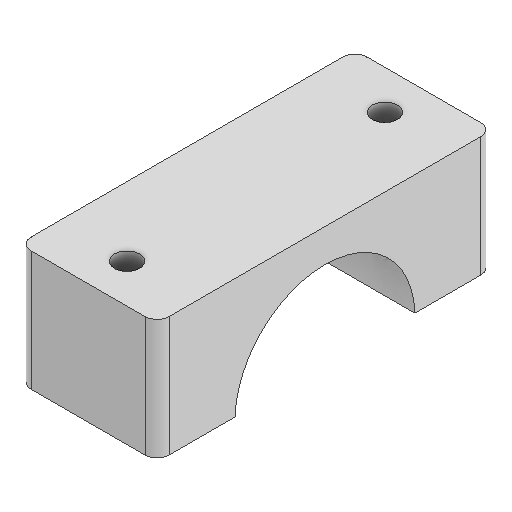
# Autodesk Inventor part: 3DP_ASA_Preamp_Case_Clamp
Saved by Autodesk Inventor 2026.1 (Build 301233000, 233)
## iProperties
Created: 2025-06-27
Part Number: 3DP_ASA_Preamp_Case_Clamp
Material: Generic
Document SubType Name: Modeling
Designer: User
Density: 1 g/cm^3
Appearance: Default
Author: User
Autodesk Inventor part; units mm, degrees
ref_plane "YZ Plane" through (0, 0, 0) normal (1, 0, 0) x (0, 1, 0)
ref_plane "XZ Plane" through (0, 0, 0) normal (0, 1, 0) x (-1, 0, 0)
ref_plane "XY Plane" through (0, 0, 0) normal (0, 0, 1) x (1, 0, 0)
sketch "Sketch1" plane through (0, 0, 0) normal (0, 1, 0) x (-1, 0, 0)
  line L0 (12.5, 25.5) -> (-12.5, 25.5)
  line L1 (-12.5, 25.5) -> (-12.5, -25.5)
  line L2 (-12.5, -25.5) -> (12.5, -25.5)
  line L3 (12.5, -25.5) -> (12.5, 25.5)
  line L4 (13, 26) -> (-13, 26)
  line L5 (-13, 26) -> (-13, -26)
  line L6 (-13, -26) -> (13, -26)
  line L7 (13, -26) -> (13, 26)
  line L8 (15, 28) -> (-15, 28)
  line L9 (-15, 28) -> (-15, -28)
  line L10 (-15, -28) -> (15, -28)
  circle A0 centre (8.5, 21.5) radius 2
  circle A1 centre (8.5, -21.5) radius 2
  circle A2 centre (-8.5, 21.5) radius 2
  circle A3 centre (-8.5, -21.5) radius 2
  line L11 (15, -28) -> (38, -28)
  line L12 (38, -28) -> (38, -26)
  line L13 (38, -26) -> (13, -26)
  line L14 (13, 26) -> (38, 26)
  line L15 (38, 26) -> (38, 28)
  line L16 (38, 28) -> (15, 28)
  line L17 (38, -26) -> (38, 26)
  line L18 (12.5, -15.5) -> (-12.5, -15.5)
  line L19 (12.5, 15.5) -> (-12.5, 15.5)
  line L20 (12.5, -15.5) -> (13, -15.5)
  line L21 (12.5, 15.5) -> (13, 15.5)
  line L22 (-12.5, -15.5) -> (-13, -15.5)
  line L23 (-12.5, 15.5) -> (-13, 15.5)
  point P0 (0, 0)
  dimension "d0" = 51
  dimension "d1" = 25
  dimension "d2" = 12.5
  dimension "d3" = 25.5
  dimension "d4" = 4
  dimension "d5" = 4
  dimension "d6" = 4
  dimension "d7" = 4
  dimension "d8" = 0.5
  dimension "d10" = 4
  dimension "d11" = 4
  dimension "d12" = 4
  dimension "d13" = 4
  dimension "d50" = 25
  dimension "d51" = 10
  dimension "d52" = 10
  constraints: 48 end point, 12 perpendicular, 8 point on line, 5 parallel, 4 centre point, 4 coincident, 3 horizontal, 2 horizontal alignment, 2 vertical alignment, 1 vertical, 5 other
  measures "d0" distance between parallel lines of L2 L0
  measures "d1" distance of L1.end L2.end
  measures "d2" distance from line of L3 point (0, 0)
  measures "d3" distance from line of L2 point (0, 0)
  measures "d4" distance from line of L0 point (8.5, 21.5)
  measures "d5" distance from line of L3 point (8.5, 21.5)
  measures "d6" distance from line of L1 point (-8.5, 21.5)
  measures "d7" distance from line of L2 point (8.5, -21.5)
  measures "d8" distance between parallel lines of L3 L7
  measures "d10" diameter of A0
  measures "d11" diameter of A1
  measures "d12" diameter of A2
  measures "d13" diameter of A3
  measures "d50" distance between parallel lines of L17 L7
  measures "d51" distance between parallel lines of L2 L18
  measures "d52" distance between parallel lines of L0 L19
extrude "Extrusion1" add sketch "Sketch1" against normal blind 10 contours L3 L19 L1 L0 | L0 L1 L23 L5 L4 L7 L21 L3 | L21 L7 L20 L3 | L3 L18 L1 L19 | L1 L22 L5 L23 | L20 L7 L6 L5 L22 L1 L2 L3 | L3 L2 L1 L18 | L7 L14 L17 L13 | L5 L6 L13 L12 L11 L10 L9 L8 L16 L15 L14 L4 | A0 | A1 | A2 | A3
extrude "Extrusion2" add sketch "Sketch1" along normal blind 7 contours L5 L6 L13 L12 L11 L10 L9 L8 L16 L15 L14 L4
extrude "Extrusion3" cut sketch "Sketch1" against normal blind 6 contours A0 | A1 | A2 | A3
extrude "Extrusion8" cut sketch "Sketch1" against normal blind 7 contours L21 L7 L20 L3 | L3 L18 L1 L19 | L1 L22 L5 L23 | L7 L14 L17 L13
fillet "Fillet3" radius 2 6 edges at (-13, -3.5, -15.5) (-13, -3.5, -26) (13, -3.5, -15.5) (13, -3.5, 15.5) (-13, -3.5, 15.5) (-13, -3.5, 26)
sketch "Sketch7" plane through (8.5, -6, -21.5) normal (0, 1, 0) x (1, 0, 0)
  circle A0 centre (0, 0) radius 2 projected
  circle A1 centre (-17, 0) radius 2 projected
  circle A2 centre (-17, -43) radius 2 projected
  circle A3 centre (0, -43) radius 2 projected
  point P0 (-8.5, -21.5)
extrude "Extrusion9" cut sketch "Sketch7" against normal blind 1
sketch "Sketch8" plane through (-38, -10, -28) normal (-1, 0, 0) x (0, 0, 1)
  line L0 (54, 17) -> (54, 3) projected
  line L1 (54, 3) -> (2, 3) projected
  line L2 (2, 3) -> (2, 17) projected
  line L3 (0, 17) -> (2, 17) projected
  line L4 (0, 17) -> (0, 0) projected
  line L5 (56, 0) -> (0, 0) projected
  line L6 (56, 0) -> (56, 17) projected
  line L7 (54, 17) -> (56, 17) projected
  line L8 (2, 17) -> (54, 17)
  line L9 (13.7, 17) -> (13.7, 9)
  line L10 (13.7, 9) -> (19.7, 9)
  line L11 (19.7, 9) -> (19.7, 17)
  line L12 (36.7, 17) -> (36.7, 9)
  line L13 (36.7, 9) -> (42.7, 9)
  line L14 (42.7, 9) -> (42.7, 17)
  point P0 (28, 10)
  dimension "d58" = 6
  dimension "d59" = 6
  dimension "d60" = 17
  dimension "d63" = 11.7
  dimension "d66" = 8
  constraints: 14 end point, 6 point on line, 4 perpendicular, 1 parallel, 1 vertical
  measures "d58" distance between parallel lines of L11 L9
  measures "d59" distance between parallel lines of L14 L12
  measures "d60" distance between parallel lines of L12 L11
  measures "d63" distance between parallel lines of L2 L9
  measures "d66" distance between parallel lines of L8 L10
extrude "Extrusion10" add sketch "Sketch8" against normal blind 2 contours L0 L1 L2 L8 L9 L10 L11 L12 L13 L14
fillet "Fillet4" radius 2 8 edges at (-37, -1, -14.3) (-37, -1, -8.3) (-37, -1, 8.7) (-37, -1, 14.7) (-38, -1.5, 28) (15, -1.5, 28) (15, -1.5, -28) (-38, -1.5, -28)
fillet "Fillet5" radius 2 2 edges at (-36, 0, -26) (-36, 0, 26)
sketch "Sketch10" plane through (0, -10, 0) normal (0, -1, 0) x (1, 0, 0)
  line L0 (-15, 26) -> (-34, 26) projected
  arc A0 (-34, 26) -> (-36, 24) centre (-34, 24) ccw projected
  line L1 (-36, -24) -> (-36, 24) projected
  arc A1 (-36, -24) -> (-34, -26) centre (-34, -24) ccw projected
  line L2 (-34, -26) -> (-15, -26) projected
  arc A2 (-38, -26) -> (-36, -28) centre (-36, -26) ccw projected
  line L3 (-36, -28) -> (13, -28) projected
  arc A3 (13, -28) -> (15, -26) centre (13, -26) ccw projected
  line L4 (15, -26) -> (15, 26) projected
  arc A4 (15, 26) -> (13, 28) centre (13, 26) ccw projected
  line L5 (13, 28) -> (-36, 28) projected
  arc A5 (-36, 28) -> (-38, 26) centre (-36, 26) ccw projected
  line L6 (-38, 26) -> (-38, -26) projected
  line L7 (-36, 24) -> (-36, 28)
  line L8 (-36, -24) -> (-36, -28)
  line L9 (-15, 28) -> (-15, -28)
  point P0 (0, 0)
  constraints: 6 end point, 3 point on line, 2 perpendicular, 1 tangent
extrude "Extrusion11" add sketch "Sketch10" along normal blind 20 contours L9 L2 A1 L1 A0 L0 | L0 A0 L7 L5 L9 | L9 L3 L8 A1 L2 | L1 L8 A2 L6 A5 L7
sketch "Sketch11" plane through (-38, 7, -8.3) normal (-1, 0, 0) x (0, 0, 1)
  line L0 (-17.7, -37) -> (-17.7, 0) projected
  line L1 (34.3, -37) -> (-17.7, -37) projected
  line L2 (34.3, 0) -> (34.3, -37) projected
  line L3 (34.3, 0) -> (23, 0) projected
  line L4 (23, 0) -> (23, -6) projected
  arc A0 (21, -8) -> (23, -6) centre (21, -6) ccw projected
  line L5 (21, -8) -> (19, -8) projected
  arc A1 (17, -6) -> (19, -8) centre (19, -6) ccw projected
  line L6 (17, -6) -> (17, 0) projected
  line L7 (17, 0) -> (0, 0) projected
  line L8 (0, 0) -> (0, -6) projected
  arc A2 (-2, -8) -> (0, -6) centre (-2, -6) ccw projected
  line L9 (-2, -8) -> (-4, -8) projected
  arc A3 (-6, -6) -> (-4, -8) centre (-4, -6) ccw projected
  line L10 (-6, -6) -> (-6, 0) projected
  line L11 (-17.7, 0) -> (-6, 0) projected
  arc A4 (23.2917, -37) -> (-6.6917, -37) centre (8.3, -37.5) ccw
  point P0 (8.3, -7)
  dimension "d71" = 52
  dimension "d72" = 26
  dimension "d73" = 0.5
  dimension "d74" = 30
  constraints: 2 point on circle, 2 point on line, 1 centre point, 1 coincident
  measures "d71" distance between parallel lines of L0 L2
  measures "d72" distance from line of L2 point (8.3, -37.5)
  measures "d73" distance from line of L1 point (8.3, -37.5)
  measures "d74" diameter of A4
extrude "Extrusion12" cut sketch "Sketch11" against normal through all contours A4 L1
fillet "Fillet6" radius 2 2 edges at (-15, -20, 28) (-15, -20, -28)
sketch "Sketch12" plane through (0, -30, 0) normal (0, -1, 0) x (1, 0, 0)
  arc A0 (-15, 26) -> (-17, 28) centre (-17, 26) ccw projected
  line L0 (-17, 28) -> (-36, 28) projected
  arc A1 (-36, 28) -> (-38, 26) centre (-36, 26) ccw projected
  line L1 (-38, 26) -> (-38, 14.9917) projected
  line L2 (-38, 14.9917) -> (-15, 14.9917) projected
  line L3 (-15, 14.9917) -> (-15, 26) projected
  arc A2 (-17, -28) -> (-15, -26) centre (-17, -26) ccw projected
  line L4 (-15, -26) -> (-15, -14.9917) projected
  line L5 (-15, -14.9917) -> (-38, -14.9917) projected
  line L6 (-38, -14.9917) -> (-38, -26) projected
  arc A3 (-38, -26) -> (-36, -28) centre (-36, -26) ccw projected
  line L7 (-36, -28) -> (-17, -28) projected
  point P0 (0, 0)
  point P1 (-26.5, 21.5)
  point P2 (-26.5, -21.5)
  dimension "d78" = 23
  dimension "d79" = 11.5
  dimension "d80" = 13.0083
  dimension "d81" = 6.5
  dimension "d82" = 6.5
  constraints: 1 vertical alignment
  measures "d78" distance between parallel lines of L1 L3
  measures "d79" distance from line of L3 point (-26.5, 21.5)
  measures "d80" distance between parallel lines of L2 L0
  measures "d81" distance from line of L0 point (-26.5, 21.5)
  measures "d82" distance from line of L7 point (-26.5, -21.5)
hole "Hole1" at (-26.5, -30, 21.5) at (-26.5, -30, -21.5) direction (0, 1, 0) diameter 4.2 end through all
sketch "Sketch13" plane through (0, 7, 0) normal (0, 1, 0) x (1, 0, 0)
  line L0 (-47.6538, 31.9961) -> (20.3258, 31.9961)
  line L1 (20.3258, 31.9961) -> (20.3258, -36.2753)
  line L2 (20.3258, -36.2753) -> (-47.6538, -36.2753)
  line L3 (-47.6538, -36.2753) -> (-47.6538, 31.9961)
  point P0 (0, 0)
  constraints: 8 end point, 2 parallel, 1 horizontal, 1 perpendicular
extrude "Extrusion13" cut sketch "Sketch13" against normal up to surface (17 mm away)
equation "\"d2\" = 0.5 * d1"
equation "\"d3\" = 0.5 * d0"
equation "\"d5\" = d4"
equation "\"d6\" = d5"
equation "\"d7\" = d4"
equation "\"d59\" = d58"
equation "\"d72\" = 0.5 * d71"
equation "\"d79\" = 0.5 * d78"
equation "\"d82\" = d81"
body "Solid1"
